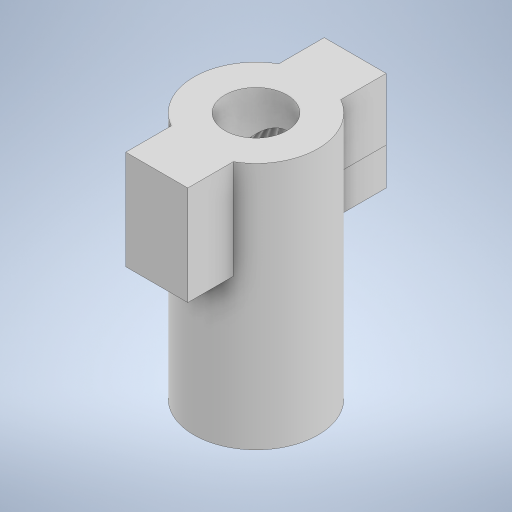
# Autodesk Inventor part: azimuth_gear_in
Saved by Autodesk Inventor 2024 (Build 280153000, 153)
## iProperties
Created: 2025-12-18
Part Number: azimuth_gear_in
Material: Generic
Document SubType Name: Modeling
Designer: schar
Density: 1 g/cm^3
Appearance: Default
Author: schar
Autodesk Inventor part; units mm, degrees
ref_plane "YZ Plane" through (0, 0, 0) normal (1, 0, 0) x (0, 1, 0)
ref_plane "XZ Plane" through (0, 0, 0) normal (0, 1, 0) x (-1, 0, 0)
ref_plane "XY Plane" through (0, 0, 0) normal (0, 0, 1) x (1, 0, 0)
sketch "Sketch1" plane through (0, 0, 0) normal (0, 1, 0) x (-1, 0, 0)
  circle A0 centre (0, 0) radius 5
  dimension "d0" = 10
  constraints: 1 centre point, 1 coincident
  measures "d0" diameter of A0
extrude "Extrusion1" add sketch "Sketch1" against normal blind 20
sketch "Sketch2" plane through (0, 0, 0) normal (1, 0, 0) x (0, 1, 0)
  line L0 (0, 0) -> (-8, 0)
  line L1 (-8, 0) -> (-8, 5)
  line L2 (-8, 5) -> (0, 5)
  line L3 (0, 5) -> (0, 0)
  line L4 (-8, 5) -> (0, 5)
  line L5 (0, 5) -> (0, 10)
  line L6 (0, 10) -> (-8, 10)
  line L7 (-8, 10) -> (-8, 5)
  line L8 (0, -5) -> (0, 5) projected
  line L9 (0, -5) -> (-8, -5)
  line L10 (-8, -5) -> (-8, -10)
  line L11 (-8, -10) -> (0, -10)
  line L12 (0, -10) -> (0, -5)
  dimension "d3" = 8
  dimension "d4" = 5
  dimension "d5" = 8
  dimension "d6" = 5
  dimension "d7" = 5
  constraints: 24 end point, 6 parallel, 3 horizontal, 3 perpendicular
  measures "d3" distance of L1.end L2.end
  measures "d4" distance of L0.end L1.end
  measures "d5" distance of L6.end L5.end
  measures "d6" distance of L5.end L4.end
  measures "d7" distance of L10.end L9.end
extrude "Extrusion2" add sketch "Sketch2" along normal mid plane 5 contours L2 L7 L6 L5 | L12 L11 L10 L9
sketch "Sketch3" plane through (-2.5, -8, 10) normal (0, 0, 1) x (1, 0, 0)
  line L0 (2.5, 0) -> (0, 0) projected
  line L1 (2.5, 8) -> (5, 8) projected
  line L2 (0, 0) -> (5, 0)
  line L3 (5, 0) -> (5, 8)
  line L4 (5, 8) -> (0, 8)
  line L5 (0, 8) -> (0, 0)
  constraints: 8 end point, 2 parallel, 1 horizontal, 1 perpendicular
extrude "Extrusion3" add sketch "Sketch3" against normal blind 20
sketch "Sketch4" plane through (0, 0, 0) normal (0, 1, 0) x (1, 0, 0)
  circle A0 centre (0, 0) radius 2.5
  dimension "d12" = 5
  constraints: 1 centre point, 1 coincident
  measures "d12" diameter of A0
extrude "Extrusion4" cut sketch "Sketch4" against normal through all
sketch "Sketch5" plane through (2.5, 0, -10) normal (0, 0, -1) x (-1, 0, 0)
  line L0 (2.5, 0) -> (2.5, -5)
  circle A0 centre (2.5, -5) radius 2.5
  line L1 (0, 0) -> (0, -20) projected
  dimension "d15" = 5
  constraints: 2 end point, 1 centre point, 1 coincident, 1 tangent, 1 vertical
  measures "d15" distance of L0.start L0.end
extrude "Extrusion5" cut sketch "Sketch5" against normal blind 10
thread "Thread1" size "M5x0.8" class "6H" standard "ANSI Metric M Profile" length 70
sketch "Sketch6" plane through (-2.5, -8, 10) normal (0, 0, 1) x (1, 0, 0)
  line L0 (0, 0) -> (5, 0) projected
  line L1 (5, 8) -> (5, 0) projected
  line L2 (0, 0) -> (5, 0)
  line L3 (5, 0) -> (5, 8)
  line L4 (5, 8) -> (0, 8)
  line L5 (0, 8) -> (0, 0)
  point P0 (2.5, 8)
  constraints: 8 end point, 2 parallel, 1 horizontal, 1 perpendicular
extrude "Extrusion6" cut sketch "Sketch6" against normal blind 2
sketch "Sketch7" plane through (2.5, 0, -10) normal (0, 0, -1) x (-1, 0, 0)
  line L0 (5, -8) -> (5, 0) projected
  line L1 (0, 0) -> (5, 0)
  line L2 (5, 0) -> (5, -8)
  line L3 (5, -8) -> (0, -8)
  line L4 (0, -8) -> (0, 0)
  point P0 (2.5, 0)
  constraints: 8 end point, 2 parallel, 1 horizontal, 1 perpendicular
extrude "Extrusion7" cut sketch "Sketch7" against normal blind 2
body "Solid1"
